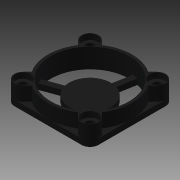
# Autodesk Inventor part: fan_3007_base
Saved by Autodesk Inventor 2013 (Build 170138000, 138)
## iProperties
Created: 2014-03-19
Part Number: fan_3007_base
Document SubType Name: Modeling
Designer: Noa Izumi
Material: Default
Density: 1 g/cm^3
Control State: 0
Master: False
Checked Out: False
Shininess: 41.0
Density: 0.0
Volumn: 0.0
Area: 0.0
PropertySet Name: Model Information
Author: Noa Izumi
Autodesk Inventor part; units mm, degrees
ref_plane "YZ Plane" through (0, 0, 0) normal (1, 0, 0) x (0, 1, 0)
ref_plane "XZ Plane" through (0, 0, 0) normal (0, 1, 0) x (-1, 0, 0)
ref_plane "XY Plane" through (0, 0, 0) normal (0, 0, 1) x (1, 0, 0)
sketch "Sketch1" plane through (0, 0, 0) normal (0, 0, 1) x (1, 0, 0)
  line L0 (0, 0) -> (30, 0)
  line L1 (30, 0) -> (30, 30)
  line L2 (30, 30) -> (0, 30)
  line L3 (0, 30) -> (0, 0)
  dimension "d0" = 30
  dimension "d1" = 30
  constraints: 8 end point, 2 parallel, 1 horizontal, 1 perpendicular
  measures "d0" distance of L0.start L0.end
  measures "d1" distance of L2.end L0.start
extrude "Extrusion1" add sketch "Sketch1" along normal blind 2
sketch "Sketch2" plane through (0, 0, 2) normal (0, 0, 1) x (1, 0, 0)
  line L0 (0, 0) -> (0, 30) projected
  line L1 (30, 0) -> (0, 0) projected
  line L2 (30, 30) -> (30, 0) projected
  line L3 (0, 30) -> (30, 30) projected
  circle A0 centre (15, 15) radius 15
  circle A1 centre (3, 27) radius 3
  circle A2 centre (3, 3) radius 3
  circle A3 centre (27, 27) radius 3
  circle A4 centre (27, 3) radius 3
  line L4 (0.8787, 5.1213) -> (24.8787, 29.1213)
  line L5 (5.1213, 0.8787) -> (29.1213, 24.8787)
  line L6 (5.1213, 29.1213) -> (29.1213, 5.1213)
  line L7 (24.8787, 0.8787) -> (0.8787, 24.8787)
  dimension "d4" = 15
  dimension "d5" = 15
  dimension "d6" = 30
  dimension "d7" = 3
  dimension "d8" = 3
  dimension "d9" = 3
  dimension "d10" = 3
  dimension "d11" = 3
  dimension "d12" = 3
  dimension "d13" = 3
  dimension "d14" = 3
  dimension "d15" = 6
  dimension "d16" = 6
  dimension "d17" = 6
  dimension "d18" = 6
  constraints: 8 end point, 8 point on circle, 5 centre point, 5 tangent, 2 parallel, 1 perpendicular
  measures "d4" horizontal distance of L0.start A0.centre
  measures "d5" horizontal distance of L0.start A0.centre
  measures "d6" diameter of A0
  measures "d7" distance from line of L0 A1.centre
  measures "d8" distance from line of A1.centre L3
  measures "d9" distance from line of L0 A2.centre
  measures "d10" distance from line of L1 A2.centre
  measures "d11" distance from line of L3 A3.centre
  measures "d12" distance from line of L2 A3.centre
  measures "d13" distance from line of L2 A4.centre
  measures "d14" distance from line of L1 A4.centre
  measures "d15" diameter of A1
  measures "d16" diameter of A3
  measures "d17" diameter of A4
  measures "d18" diameter of A2
extrude "Extrusion2" add sketch "Sketch2" along normal blind 5 contours A2 A0 | A0 L7 L4 | L4 A0 A2 | A0 L5 L7 | A2 A0 L5 | A1 A0 | L7 A1 A0 | A0 A1 L6 L4 L7 | L4 L7 L5 A0 A2 | A2 A0 | A4 A0 | L7 L5 L6 A0 A4 | A0 A4 L7 | A0 A1 | L4 L6 L5 L7 | A4 A0 | A0 L4 L6 | L6 A0 A1 | L4 A0 A3 L5 L6 | A0 L6 L5 | A4 A0 L6 | A3 A0 | L4 A3 A0 | A0 A3 L5 | A0 A3
sketch "Sketch3" plane through (0, 0, 7) normal (0, 0, 1) x (1, 0, 0)
  arc A0 (5.1213, 29.1213) -> (0.8787, 24.8787) centre (3, 27) ccw projected
  arc A1 (0.8787, 5.1213) -> (5.1213, 0.8787) centre (3, 3) ccw projected
  arc A2 (24.8787, 0.8787) -> (29.1213, 5.1213) centre (27, 3) ccw projected
  arc A3 (29.1213, 24.8787) -> (24.8787, 29.1213) centre (27, 27) ccw projected
  constraints: 4 coincident
hole "Hole1" at (3, 27, 7) at (27, 27, 7) at (27, 3, 7) at (3, 3, 7) direction (0, 0, -1) diameter 3 end through all
fillet "Fillet1" radius 3 4 edges at (0, 0, 1) (30, 0, 1) (30, 30, 1) (0, 30, 1)
sketch "Sketch4" plane through (0, 0, 7) normal (0, 0, 1) x (1, 0, 0)
  arc A0 (5.1213, 29.1213) -> (0.8787, 24.8787) centre (3, 27) ccw projected
  arc A1 (0.8787, 5.1213) -> (5.1213, 0.8787) centre (3, 3) ccw projected
  arc A2 (24.8787, 0.8787) -> (29.1213, 5.1213) centre (27, 3) ccw projected
  arc A3 (29.1213, 24.8787) -> (24.8787, 29.1213) centre (27, 27) ccw projected
  constraints: 4 coincident
hole "Hole2" at (3, 3, 7) at (27, 3, 7) at (3, 27, 7) at (27, 27, 7) direction (0, 0, -1) diameter 5.6 depth 2
sketch "Sketch5" plane through (0, 0, 7) normal (0, 0, 1) x (1, 0, 0)
  arc A0 (27.5136, 6.729) -> (27.5136, 23.271) centre (15, 15) ccw projected
  circle A1 centre (15, 15) radius 14
  dimension "d36" = 28
  constraints: 1 centre point, 1 coincident
  measures "d36" diameter of A1
extrude "Extrusion3" cut sketch "Sketch5" against normal blind 5
sketch "Sketch6" plane through (15, 15, 2) normal (0, 0, 1) x (1, 0, 0)
  circle A0 centre (0, 0) radius 14 projected
  line L0 (-13.4641, -3.8364) -> (-7.3268, -1.6026)
  line L1 (-6.6427, -3.4819) -> (-12.7801, -5.7157)
  line L2 (0.3059, 7.4938) -> (1.4401, 13.9257)
  line L3 (3.4097, 13.5784) -> (2.2755, 7.1465)
  line L4 (6.3368, -4.0118) -> (11.34, -8.21)
  line L5 (10.0544, -9.7421) -> (5.0512, -5.5439)
  arc A1 (-6.6427, -3.4819) -> (5.0512, -5.5439) centre (0, 0) ccw
  arc A2 (6.3368, -4.0118) -> (2.2755, 7.1465) centre (0, 0) ccw
  arc A3 (0.3059, 7.4938) -> (-7.3268, -1.6026) centre (0, 0) ccw
  arc A4 (-12.7801, -5.7157) -> (10.0544, -9.7421) centre (0, 0) ccw
  arc A5 (11.34, -8.21) -> (3.4097, 13.5784) centre (0, 0) ccw
  arc A6 (1.4401, 13.9257) -> (-13.4641, -3.8364) centre (0, 0) ccw
  constraints: 12 end point, 12 point on circle, 6 centre point, 3 parallel, 1 coincident, 1 point on line, 2 other
extrude "Extrusion4" cut sketch "Sketch6" against normal through all contours A0 L4 A2 L3 | L2 A3 L0 A0 | A0 L1 A1 L5
